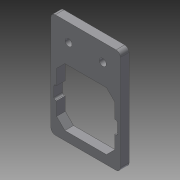
# Autodesk Inventor part: Motor_Clamp
Saved by Autodesk Inventor 2015 (Build 190159000, 159)
## iProperties
Created: 2015-01-10
Part Number: Motor_Clamp
Material: Generic
Document SubType Name: Modeling
Designer: Drew
Density: 1 g/cm^3
Appearance: Default
Author: Drew
Autodesk Inventor part; units mm, degrees
ref_plane "YZ Plane" through (0, 0, 0) normal (1, 0, 0) x (0, 1, 0)
ref_plane "XZ Plane" through (0, 0, 0) normal (0, 1, 0) x (-1, 0, 0)
ref_plane "XY Plane" through (0, 0, 0) normal (0, 0, 1) x (1, 0, 0)
sketch "Sketch1" plane through (0, 0, 0) normal (0, 0, 1) x (1, 0, 0)
  line L0 (-25.4, 45.4025) -> (-25.4, -24.4475)
  line L1 (-22.225, -27.6225) -> (22.225, -27.6225)
  line L2 (25.4, -24.4475) -> (25.4, 45.4025)
  line L3 (22.225, 48.5775) -> (-22.225, 48.5775)
  line L4 (0, 57.3133) -> (0, -29.6676)
  circle A0 centre (-12.5413, 35.8775) radius 2.54
  circle A1 centre (12.5412, 35.8775) radius 2.54
  arc A2 (-25.4, -24.4475) -> (-22.225, -27.6225) centre (-22.225, -24.4475) ccw
  arc A3 (22.225, -27.6225) -> (25.4, -24.4475) centre (22.225, -24.4475) ccw
  arc A4 (25.4, 45.4025) -> (22.225, 48.5775) centre (22.225, 45.4025) ccw
  arc A5 (-22.225, 48.5775) -> (-25.4, 45.4025) centre (-22.225, 45.4025) ccw
  line L5 (-55.0388, 0) -> (75.1356, 0)
  point P0 (-25.4, 48.5775)
  point P1 (-25.4, -27.6225)
  point P2 (25.4, -27.6225)
  point P3 (25.4, 48.5775)
  dimension "d10" = 50.8
  dimension "d11" = 76.2
  dimension "d12" = 5.08
  dimension "d13" = 25.0825
  dimension "d18" = 3.175
  constraints: 12 end point, 8 point on circle, 8 point on line, 8 tangent, 6 centre point, 3 equal radius, 3 vertical, 2 perpendicular, 1 horizontal, 1 symmetric about line, 2 other
  measures "d10" distance of point (25.4, 48.577) point (-25.4, 48.577)
  measures "d11" distance between parallel lines of L1 L3
  measures "d12" diameter of A0
  measures "d13" distance of A1.centre A0.centre
  measures "d18" radius of A2
extrude "Extrusion2" add sketch "Sketch1" along normal blind 6.35
sketch "Sketch2" plane through (0, 0, 6.35) normal (0, 0, 1) x (1, 0, 0)
  line L0 (15.209, -21.209) -> (-15.209, -21.209)
  line L1 (-21.209, -15.209) -> (-21.209, 15.209)
  line L2 (-15.209, 21.209) -> (15.209, 21.209)
  line L3 (21.209, 15.209) -> (21.209, -15.209)
  line L4 (21.209, -21.209) -> (-21.209, 21.209) construction
  line L5 (-21.209, -21.209) -> (21.209, 21.209) construction
  line L6 (-21.209, 15.209) -> (-15.209, 21.209)
  line L7 (21.209, 15.209) -> (15.209, 21.209)
  line L8 (21.209, -15.209) -> (15.209, -21.209)
  line L9 (-15.209, -21.209) -> (-21.209, -15.209)
  point P0 (0, 0)
  dimension "d24" = 42.418
  dimension "d25" = 42.418
  dimension "d26" = 6
  dimension "d27" = 6
  dimension "d28" = 6
  dimension "d29" = 6
  dimension "d30" = 6
  dimension "d31" = 6
  dimension "d32" = 6
  dimension "d33" = 6
  constraints: 20 end point, 8 point on line, 2 midpoint, 2 parallel, 1 horizontal, 1 perpendicular
  measures "d24" distance of L4.end L5.end
  measures "d25" distance of L5.start L4.end
  measures "d26" distance of L1.end L4.end
  measures "d27" distance of L2.start L4.end
  measures "d28" distance of L3.start L5.end
  measures "d29" distance of L2.end L5.end
  measures "d30" distance of L3.end L4.start
  measures "d31" distance of L0.start L4.start
  measures "d32" distance of L0.end L5.start
  measures "d33" distance of L1.start L5.start
extrude "Extrusion3" cut sketch "Sketch2" against normal up to next
sketch "Sketch3" plane through (0, 0, 6.35) normal (0, 0, 1) x (1, 0, 0)
  line L0 (0, 74.5248) -> (0, -62.4529)
  line L1 (-21.209, 4.2436) -> (-23.241, 4.2436)
  line L2 (-23.241, 4.2436) -> (-23.241, -5.3802)
  line L3 (-23.241, -5.3802) -> (-21.209, -5.3802)
  line L4 (-21.209, -5.3802) -> (-21.209, 4.2436)
  line L5 (-21.209, 15.209) -> (-21.209, -15.209) projected
  line L6 (21.209, 4.2436) -> (23.241, 4.2436)
  line L7 (23.241, 4.2436) -> (23.241, -5.3802)
  line L8 (23.241, -5.3802) -> (21.209, -5.3802)
  line L9 (21.209, -5.3802) -> (21.209, 4.2436)
  point P0 (0, 0)
  point P1 (-21.209, 0)
  point P2 (21.209, 0)
  dimension "d39" = 2.032
  constraints: 18 end point, 5 symmetric about line, 2 perpendicular, 2 point on line, 1 collinear, 1 horizontal, 1 midpoint, 1 vertical
  measures "d39" distance of L1.start L1.end
extrude "Extrusion4" cut sketch "Sketch3" against normal up to next
fillet "Fillet1" radius 1.27 4 edges at (-23.241, 4.2436, 3.175) (-23.241, -5.3802, 3.175) (23.241, 4.2436, 3.175) (23.241, -5.3802, 3.175)
equation "\"d25\" = d24"
equation "\"d27\" = d26"
equation "\"d28\" = d26"
equation "\"d29\" = d28"
equation "\"d30\" = d26"
equation "\"d31\" = d30"
equation "\"d32\" = d26"
equation "\"d33\" = d32"
body "Solid2"
